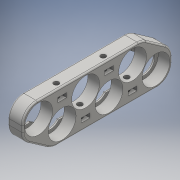
# Autodesk Inventor part: BatteryHolder2P
Saved by Autodesk Inventor 2016 (Build 200138000, 138)
## iProperties
Created: 2026-04-29
Part Number: BatteryHolder2P
Material: Generic
Document SubType Name: Modeling
Designer: Steve
Density: 1 g/cm^3
Appearance: Default
Author: Steve
Autodesk Inventor part; units mm, degrees
ref_plane "YZ Plane" through (0, 0, 0) normal (1, 0, 0) x (0, 1, 0)
ref_plane "XZ Plane" through (0, 0, 0) normal (0, 1, 0) x (-1, 0, 0)
ref_plane "XY Plane" through (0, 0, 0) normal (0, 0, 1) x (1, 0, 0)
sketch "Sketch4" plane through (0, 0, 0) normal (1, 0, 0) x (0, 1, 0)
  circle A0 centre (0, -11) radius 9.5
  circle A1 centre (-16, 0) radius 9.5
  circle A2 centre (-48, 0) radius 9.5
  circle A3 centre (-80, 0) radius 9.5
  circle A4 centre (-32, -11) radius 9.5
  circle A5 centre (-64, -11) radius 9.5
  line L0 (-91, -8) -> (-71, -22)
  line L1 (-91, -8) -> (-91, 11)
  circle A6 centre (-80, 0) radius 7.25
  circle A7 centre (-64, -11) radius 7.25
  circle A8 centre (-48, 0) radius 7.25
  circle A9 centre (-16, 0) radius 7.25
  circle A10 centre (0, -11) radius 7.25
  circle A11 centre (-32, -11) radius 7.25
  line L2 (11, -3) -> (-9, 11)
  line L3 (11, -22) -> (11, -3)
  line L4 (-9, 11) -> (-91, 11)
  line L5 (11, -22) -> (-71, -22)
  point P0 (0, 0)
  point P1 (0, 0)
  dimension "d543" = 90
  dimension "d545" = 90
  dimension "d546" = 124.992
  dimension "d547" = 124.992
  dimension "d548" = 145.008
  dimension "d550" = 11
  dimension "d551" = 11
  dimension "d552" = 11
  dimension "d553" = 11
  dimension "d554" = 11
  dimension "d555" = 16
  dimension "d556" = 16
  dimension "d557" = 16
  dimension "d558" = 16
  dimension "d559" = 16
  dimension "d560" = 11
  dimension "d561" = 11
  dimension "d562" = 11
  dimension "d580" = 80
  dimension "d612" = 19
  dimension "d613" = 19
  dimension "d614" = 82
  dimension "d615" = 82
  dimension "d638" = 14.5
  dimension "d639" = 19
  dimension "d640" = 19
  dimension "d641" = 19
  dimension "d642" = 19
  dimension "d643" = 19
  dimension "d644" = 19
  constraints: 12 centre point, 12 end point, 6 coincident, 1 horizontal, 1 vertical
  measures "d543" angle of L4 L1
  measures "d545" angle of L3 L5
  measures "d546" angle of L1 L0
  measures "d547" angle of L3 L2
  measures "d548" angle of L2 L4
  measures "d550" distance of point (0, 0) A0.centre
  measures "d551" vertical distance of A11.centre point (0, 0)
  measures "d552" vertical distance of A5.centre point (0, 0)
  measures "d553" distance from line of L5 A0.centre
  measures "d554" distance from line of L4 A1.centre
  measures "d555" horizontal distance of A5.centre A3.centre
  measures "d556" horizontal distance of A2.centre A7.centre
  measures "d557" horizontal distance of A4.centre A2.centre
  measures "d558" horizontal distance of A1.centre A4.centre
  measures "d559" horizontal distance of A0.centre A1.centre
  measures "d560" distance from line of L3 A0.centre
  measures "d561" distance from line of L1 A3.centre
  measures "d562" distance from line of L4 A3.centre
  measures "d580" distance of point (0, 0) A6.centre
  measures "d612" distance of L0.start L1.end
  measures "d613" distance of L3.start L2.start
  measures "d614" distance of L2.end L1.end
  measures "d615" distance of L3.start L0.end
  measures "d638" diameter of A6
  measures "d639" diameter of A3
  measures "d640" diameter of A5
  measures "d641" diameter of A2
  measures "d642" diameter of A4
  measures "d643" diameter of A1
  measures "d644" diameter of A0
sketch "Sketch5" plane through (0, 0, 0) normal (1, 0, 0) x (0, 1, 0)
  line L0 (-82.5494, -3.7082) -> (-66.5494, -14.7082)
  line L1 (-77.4506, 3.7082) -> (-61.4506, -7.2918)
  line L2 (4.5, -22) -> (-4.5, -22)
  line L3 (-4.5, -22) -> (-4.5, -16)
  line L4 (4.5, -16) -> (4.5, -22)
  line L5 (-82.5494, -3.7082) -> (-66.5494, -14.7082)
  line L6 (-77.4506, 3.7082) -> (-61.4506, -7.2918)
  line L7 (-66.5494, -5.5) -> (3.3859, -5.5)
  line L8 (3.3859, -5.5) -> (3.3859, -15.5)
  line L9 (3.3859, -15.5) -> (-66.5494, -15.5)
  line L10 (-66.5494, -15.5) -> (-66.5494, -5.5)
  line L11 (-83.8188, -5.5) -> (-83.8188, 4.5)
  line L12 (-27.5, -22) -> (-36.5, -22)
  line L13 (-36.5, -22) -> (-36.5, -16)
  line L14 (-36.5, -16) -> (-27.5, -16)
  line L15 (-27.5, -16) -> (-27.5, -22)
  line L16 (-59.5, -22) -> (-68.5, -22)
  line L17 (-68.5, -22) -> (-68.5, -16)
  line L18 (-68.5, -16) -> (-59.5, -16)
  line L19 (-59.5, -16) -> (-59.5, -22)
  line L20 (-2.5494, -14.7082) -> (-18.5494, -3.7082)
  line L21 (2.5494, -7.2918) -> (-13.4506, 3.7082)
  line L22 (-2.5494, -14.7082) -> (2.5494, -7.2918)
  line L23 (-13.4506, 3.7082) -> (-18.5494, -3.7082)
  line L24 (-82.5494, -3.7082) -> (-77.4506, 3.7082)
  line L25 (-61.4506, -7.2918) -> (-66.5494, -14.7082)
  line L26 (-19.0938, 4.5) -> (-19.0938, -5.5)
  line L27 (-19.0938, 4.5) -> (-83.8188, 4.5)
  line L28 (-83.8188, -5.5) -> (-19.0938, -5.5)
  line L29 (-50.5494, -3.7082) -> (-34.5494, -14.7082)
  line L30 (-45.4506, 3.7082) -> (-29.4506, -7.2918)
  line L31 (-29.4506, -7.2918) -> (-34.5494, -14.7082)
  line L32 (-50.5494, -3.7082) -> (-45.4506, 3.7082)
  line L33 (-84.5, 11) -> (-75.5, 11)
  line L34 (-75.5, 11) -> (-75.5, 5)
  line L35 (-75.5, 5) -> (-84.5, 5)
  line L36 (-84.5, 5) -> (-84.5, 11)
  line L37 (-52.5, 11) -> (-43.5, 11)
  line L38 (-43.5, 11) -> (-43.5, 5)
  line L39 (-43.5, 5) -> (-52.5, 5)
  line L40 (-52.5, 5) -> (-52.5, 11)
  line L41 (-20.5, 11) -> (-11.5, 11)
  line L42 (-11.5, 11) -> (-11.5, 5)
  line L43 (-11.5, 5) -> (-20.5, 5)
  line L44 (-20.5, 5) -> (-20.5, 11)
  line L45 (-4.5, -16) -> (4.5, -16)
  point P0 (0, 0)
  point P1 (0, 0)
  point P2 (0, 0)
  dimension "d538" = 11
  dimension "d563" = 11
  dimension "d564" = 11
  dimension "d565" = 22
  dimension "d566" = 22
  dimension "d567" = 22
  dimension "d568" = 6
  dimension "d569" = 6
  dimension "d570" = 6
  dimension "d571" = 6
  dimension "d572" = 4.5
  dimension "d573" = 9
  dimension "d574" = 9
  dimension "d575" = 9
  dimension "d576" = 9
  dimension "d577" = 6
  dimension "d578" = 23
  dimension "d579" = 23
  dimension "d581" = 75.5
  dimension "d582" = 23
  dimension "d583" = 23
  dimension "d591" = 4.5
  dimension "d592" = 15.5
  dimension "d593" = 10
  dimension "d594" = 10
  constraints: 92 end point, 17 parallel, 10 perpendicular, 9 horizontal, 3 point on line, 1 collinear
  measures "d538" distance from line of L41 point (0, 0)
  measures "d563" distance from line of point (0, 0) L33
  measures "d564" distance from line of point (0, 0) L37
  measures "d565" distance from line of point (0, 0) L2
  measures "d566" distance from line of point (0, 0) L12
  measures "d567" distance from line of point (0, 0) L16
  measures "d568" distance between parallel lines of L2 L45
  measures "d569" distance between parallel lines of L12 L14
  measures "d570" distance between parallel lines of L35 L33
  measures "d571" distance between parallel lines of L39 L37
  measures "d572" distance from line of point (0, 0) L4
  measures "d573" distance between parallel lines of L3 L4
  measures "d574" distance between parallel lines of L44 L42
  measures "d575" distance between parallel lines of L40 L38
  measures "d576" distance between parallel lines of L36 L34
  measures "d577" distance of L43.end L41.start
  measures "d578" distance between parallel lines of L15 L3
  measures "d579" distance between parallel lines of L19 L13
  measures "d581" distance from line of point (0, 0) L34
  measures "d582" distance between parallel lines of L40 L34
  measures "d583" distance between parallel lines of L44 L38
  measures "d591" distance from line of point (0, 0) L27
  measures "d592" distance from line of point (0, 0) L9
  measures "d593" distance of L11.start L11.end
  measures "d594" distance of L7.end L8.end
extrude "Extrusion11" add sketch "Sketch4" along normal blind 10 contours L1 L4 L2 L3 L5 L0
extrude "Extrusion12" add sketch "Sketch4" along normal blind 2 contours A0 | A1 | A2 | A3 | A4 | A5
extrude "Extrusion13" cut sketch "Sketch5" along normal blind 2 contours L24 L1 L7 L28 L0 | L0 L28 L11 L27 L26 L7 L30 L32 L29 L1 L24 | L28 L10 L0 | L25 L1 L7 L29 L31 L30 L20 L22 L21 L8 L9 L10 | L10 L7 L1 L25 | L29 L32 L30 L7 | L7 L30 L31 L29 | L21 L22 L20 L7 | L7 L20 L23 L21
sketch "Sketch6" plane through (0, -71, -22) normal (0, 0, -1) x (-1, 0, 0)
  circle A0 centre (-6, 55) radius 1.75
  circle A1 centre (-6, 23) radius 1.75
  line L0 (0, 82) -> (-10, 82) projected
  line L1 (0, 0) -> (0, 82) projected
  point P0 (0, 71)
  dimension "d595" = 3.5
  dimension "d596" = 3.5
  dimension "d597" = 27
  dimension "d598" = 32
  dimension "d599" = 6
  dimension "d600" = 6
  constraints: 2 centre point
  measures "d595" diameter of A0
  measures "d596" diameter of A1
  measures "d597" distance from line of L0 A0.centre
  measures "d598" distance of A1.centre A0.centre
  measures "d599" distance from line of L1 A0.centre
  measures "d600" distance from line of L1 A1.centre
extrude "Extrusion14" cut sketch "Sketch6" against normal blind 15
sketch "Sketch7" plane through (0, -91, 11) normal (0, 0, 1) x (1, 0, 0)
  circle A0 centre (6, 59) radius 1.75
  circle A1 centre (6, 27) radius 1.75
  line L0 (0, 82) -> (0, 0) projected
  line L1 (0, 0) -> (10, 0) projected
  point P0 (0, 91)
  dimension "d603" = 3.5
  dimension "d604" = 3.5
  dimension "d605" = 6
  dimension "d606" = 6
  dimension "d607" = 27
  dimension "d608" = 32
  constraints: 2 centre point
  measures "d603" diameter of A0
  measures "d604" diameter of A1
  measures "d605" distance from line of L0 A1.centre
  measures "d606" distance from line of L0 A0.centre
  measures "d607" distance from line of L1 A1.centre
  measures "d608" distance of A0.centre A1.centre
extrude "Extrusion15" cut sketch "Sketch7" against normal blind 15
fillet "Fillet3" radius 10 6 edges at (5, -91, 11) (5, 11, -22) (5, 11, -3) (5, -9, 11) (5, -91, -8) (5, -71, -22)
sketch "Sketch8" plane through (10, 0, 0) normal (1, 0, 0) x (0, 0, -1)
  line L0 (17, -51) -> (14, -51)
  line L1 (14, -51) -> (14, -45)
  line L2 (14, -45) -> (17, -45)
  line L3 (17, -45) -> (17, -51)
  line L4 (17, -19) -> (14, -19)
  line L5 (14, -19) -> (14, -13)
  line L6 (14, -13) -> (17, -13)
  line L7 (17, -13) -> (17, -19)
  line L8 (-3, -29) -> (-6, -29)
  line L9 (-6, -29) -> (-6, -35)
  line L10 (-6, -35) -> (-3, -35)
  line L11 (-3, -35) -> (-3, -29)
  line L12 (-3, -61) -> (-6, -61)
  line L13 (-6, -61) -> (-6, -67)
  line L14 (-6, -67) -> (-3, -67)
  line L15 (-3, -67) -> (-3, -61)
  line L16 (22, -67.8478) -> (22, 1) projected
  line L17 (-11, -12.1522) -> (-11, -81) projected
  line L18 (12, 11) -> (8.2066, 11) projected
  point P0 (0, 0)
  point P1 (-1, -91)
  dimension "d616" = 3
  dimension "d617" = 6
  dimension "d618" = 3
  dimension "d619" = 6
  dimension "d620" = 3
  dimension "d621" = 6
  dimension "d622" = 3
  dimension "d623" = 6
  dimension "d624" = 5
  dimension "d625" = 5
  dimension "d626" = 5
  dimension "d627" = 5
  dimension "d628" = 24
  dimension "d629" = 26
  dimension "d630" = 26
  dimension "d631" = 24
  constraints: 32 end point, 8 parallel, 4 horizontal, 4 perpendicular, 1 point on line
  measures "d616" distance of L1.end L2.end
  measures "d617" distance of L0.end L1.end
  measures "d618" distance of L5.end L6.end
  measures "d619" distance of L4.end L5.end
  measures "d620" distance of L10.end L9.end
  measures "d621" distance of L9.end L8.end
  measures "d622" distance of L14.end L13.end
  measures "d623" distance of L13.end L12.end
  measures "d624" distance between parallel lines of L16 L7
  measures "d625" distance between parallel lines of L16 L3
  measures "d626" distance between parallel lines of L17 L9
  measures "d627" distance between parallel lines of L17 L13
  measures "d628" distance from line of point (-1, -91) L14
  measures "d629" distance between parallel lines of L12 L10
  measures "d630" distance between parallel lines of L2 L4
  measures "d631" distance between parallel lines of L18 L6
extrude "Extrusion16" cut sketch "Sketch8" against normal blind 7
fillet "Fillet4" radius 1 36 edges at (0, -88.0711, 8.0711) (0, -91, -0.8967) (0, -89.8698, -7.4115) (0, -80.1585, -15.589) (0, -70.8542, -21.5374) (0, -33.4239, -22) (0, 8.0711, -19.0711) (0, 11, -10.1033) (0, 9.8698, -3.5885) (0, 0.1585, 4.589) (0, -9.1458, 10.5374) (0, -46.5761, 11) (10, -88.0711, 8.0711) (10, -91, -0.8967) (10, -89.8698, -7.4115) (10, -80.1585, -15.589) (10, -70.8542, -21.5374) (10, -33.4239, -22) (10, 8.0711, -19.0711) (10, 11, -10.1033) (10, 9.8698, -3.5885) (10, 0.1585, 4.589) (10, -9.1458, 10.5374) (10, -46.5761, 11) (0, -64, 4.5) (0, -32, 4.5) (0, -48, 7.25) (0, -13.8496, 6.9237) (0, -5.4506, -1.7918) (0, 6.9237, -13.1504) (0, -16, -15.5) (0, -48, -15.5) (0, -32, -18.25) (0, -66.1504, -17.9237) (0, -74.5494, -9.2082) (0, -86.9237, 2.1504)
body "Solid4"
